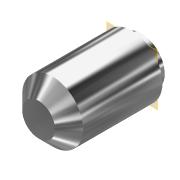
# Autodesk Inventor part: 00_Microscope_Objective
Saved by Autodesk Inventor 2019 (Build 230136000, 136)
## iProperties
Created: 2019-05-02
Part Number: 00_Microscope_Objective
Material: Generic
Document SubType Name: Modeling
Designer: diederichbenedict
Density: 1 g/cm^3
Appearance: Chrome - Polished
Author: diederichbenedict
Autodesk Inventor part; units mm, degrees
ref_plane "YZ Plane" through (0, 0, 0) normal (1, 0, 0) x (0, 1, 0)
ref_plane "XZ Plane" through (0, 0, 0) normal (0, 1, 0) x (-1, 0, 0)
ref_plane "XY Plane" through (0, 0, 0) normal (0, 0, 1) x (1, 0, 0)
ref_plane "Work Plane3" through (0, 0, 30) normal (0, 0, 1) x (1, 0, 0)
sketch "Sketch2" plane through (0, 0, 30) normal (0, 0, 1) x (1, 0, 0)
  arc A0 (80, 65) -> (65, 80) centre (65, 65) ccw projected
  line L0 (80, 65) -> (80, -65) projected
  arc A1 (65, -80) -> (80, -65) centre (65, -65) ccw projected
  line L1 (65, -80) -> (-65, -80) projected
  arc A2 (-80, -65) -> (-65, -80) centre (-65, -65) ccw projected
  line L2 (-80, -65) -> (-80, 65) projected
  arc A3 (-65, 80) -> (-80, 65) centre (-65, 65) ccw projected
  line L3 (-65, 80) -> (65, 80) projected
  line L4 (-150, -150) -> (150, -150) projected
  line L5 (150, -150) -> (150, 150) projected
  line L6 (150, 150) -> (-150, 150) projected
  line L7 (-150, 150) -> (-150, -150) projected
  circle A4 centre (0, 0) radius 13
  circle A5 centre (-67, -107.5) radius 1.95 projected
  circle A6 centre (67, 107.5) radius 1.95 projected
  circle A7 centre (-67, 107.5) radius 1.95 projected
  circle A8 centre (67, -107.5) radius 1.95 projected
  dimension "d0" = 26
  constraints: 1 centre point, 1 coincident
  measures "d0" diameter of A4
extrude "Extrusion1" add sketch "Sketch2" along normal blind 40 contours A4
chamfer "Chamfer2" distance 6 angle 45 1 edges at (-13, 0, 70)
sketch "Sketch3" plane through (0, 0, 30) normal (0, 0, -1) x (-1, 0, 0)
  circle A0 centre (0, 0) radius 13 projected
  circle A1 centre (0, 0) radius 10
  dimension "d9" = 20
  constraints: 1 centre point, 1 coincident
  measures "d9" diameter of A1
extrude "Extrusion2" add sketch "Sketch3" along normal blind 4 contours A1
body "Solid1"
